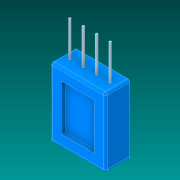
# Autodesk Inventor part: DHT11
Saved by Autodesk Inventor 2019 (Build 230136000, 136)
## iProperties
Created: 2024-01-01
Part Number: DHT11
Material: Generic
Document SubType Name: Modeling
Designer: Familia CS
Density: 1 g/cm^3
Appearance: Default
Author: Familia CS
Autodesk Inventor part; units mm, degrees
ref_plane "YZ Plane" through (0, 0, 0) normal (1, 0, 0) x (0, 1, 0)
ref_plane "XZ Plane" through (0, 0, 0) normal (0, 1, 0) x (-1, 0, 0)
ref_plane "XY Plane" through (0, 0, 0) normal (0, 0, 1) x (1, 0, 0)
sketch "Sketch1" plane through (0, 0, 0) normal (0, 0, 1) x (1, 0, 0)
  line L0 (0, 0) -> (12.5, 0)
  line L1 (12.5, 0) -> (12.5, 15.5)
  line L2 (12.5, 15.5) -> (0, 15.5)
  line L3 (0, 15.5) -> (0, 0)
  dimension "d0" = 12.5
  dimension "d1" = 15.5
  constraints: 8 end point, 2 parallel, 1 horizontal, 1 perpendicular
  measures "d0" distance of L2.end L1.end
  measures "d1" distance of L1.end L0.end
extrude "Extrusion1" add sketch "Sketch1" along normal blind 5.5
sketch "Sketch2" plane through (0, 15.5, 0) normal (0, 1, 0) x (1, 0, 0)
  circle A0 centre (10.81, -2.75) radius 0.25
  circle A1 centre (7.77, -2.75) radius 0.25
  circle A2 centre (4.73, -2.75) radius 0.25
  circle A3 centre (1.69, -2.75) radius 0.25
  point P0 (0, -5.5)
  point P1 (12.5, 0)
  dimension "d27" = 0.5
  dimension "d28" = 0.5
  dimension "d29" = 0.5
  dimension "d30" = 0.5
  constraints: 4 centre point
  measures "d27" diameter of A0
  measures "d28" diameter of A1
  measures "d29" diameter of A2
  measures "d30" diameter of A3
extrude "Extrusion2" add sketch "Sketch2" along normal blind 8
fillet "Fillet1" radius 0.5 8 edges at (0, 7.75, 5.5) (0, 0, 2.75) (6.25, 0, 5.5) (12.5, 7.75, 5.5) (6.25, 15.5, 5.5) (0, 15.5, 2.75) (12.5, 15.5, 2.75) (12.5, 0, 2.75)
sketch "Sketch3" plane through (0, 0, 5.5) normal (0, 0, 1) x (1, 0, 0)
  line L0 (2.5, 2.5) -> (10, 2.5)
  line L1 (10, 2.5) -> (10, 13)
  line L2 (10, 13) -> (2.5, 13)
  line L3 (2.5, 13) -> (2.5, 2.5)
  point P0 (0, 0)
  point P1 (12, 0.5)
  point P2 (0.5, 15)
  constraints: 8 end point, 2 parallel, 1 perpendicular
extrude "Extrusion3" cut sketch "Sketch3" against normal blind 1
body "Solid1"
